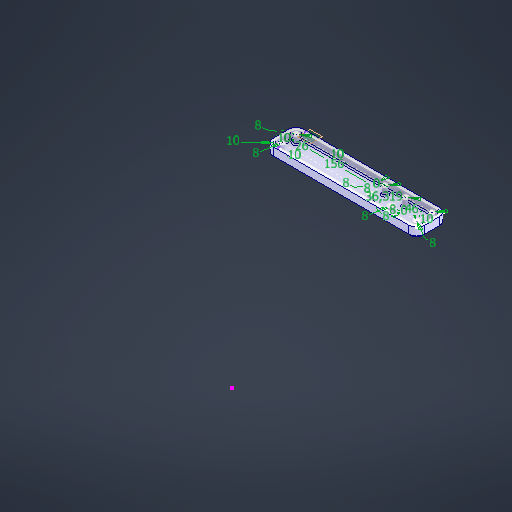
# Autodesk Inventor part: seitliche_Abdeckung_Kabel
Saved by Autodesk Inventor 2026.1 (Build 301233020, 233B)
## iProperties
Created: 2026-03-07
Part Number: seitliche_Abdeckung_Kabel
Material: Generisch
Document SubType Name: Modeling
Designer: neume
Density: 1 g/cm^3
Appearance: Vorgabe
Source: unknown
Author: neume
Autodesk Inventor part; units mm, degrees
ref_plane "YZ Plane" through (0, 0, 0) normal (1, 0, 0) x (0, 1, 0)
ref_plane "XZ Plane" through (0, 0, 0) normal (0, 1, 0) x (-1, 0, 0)
ref_plane "XY Plane" through (0, 0, 0) normal (0, 0, 1) x (1, 0, 0)
ref_plane "Arbeitsebene1" through (-314.8829, -4.3915, -452.3743) normal (0, -1, 0) x (1, 0, 0)
sketch "Skizze1" plane through (-314.8829, -4.3915, -452.3743) normal (0, -1, 0) x (1, 0, 0)
  line L0 (-16.319, 44) -> (222, 44)
  line L1 (232, 34) -> (232, 8)
  line L2 (222, -2) -> (-16.319, -2)
  line L3 (-16.319, 34) -> (139.681, 34) construction
  line L4 (139.681, 34) -> (139.681, 8) construction
  line L5 (139.681, 8) -> (-16.319, 8) construction
  line L6 (-16.319, 8) -> (-16.319, 34) construction
  circle A0 centre (-16.319, 34) radius 4
  circle A1 centre (-16.319, 8) radius 4
  circle A2 centre (139.681, 8) radius 4
  circle A3 centre (139.681, 34) radius 4
  line L7 (176, 34) -> (222, 34) construction
  line L8 (222, 34) -> (222, 8) construction
  line L9 (222, 8) -> (176, 8) construction
  line L10 (176, 8) -> (176, 34) construction
  circle A4 centre (176, 34) radius 4
  circle A5 centre (176, 8) radius 4
  circle A6 centre (222, 8) radius 4
  circle A7 centre (222, 34) radius 4
  arc A8 (-16.319, 44) -> (-26.319, 34) centre (-16.319, 34) ccw
  arc A9 (-26.319, 8) -> (-16.319, -2) centre (-16.319, 8) ccw
  arc A10 (222, -2) -> (232, 8) centre (222, 8) ccw
  arc A11 (232, 34) -> (222, 44) centre (222, 34) ccw
  line L11 (-26.319, 34) -> (-26.319, 8)
  point P0 (314.8829, 452.3743)
  point P1 (-10, 44)
  point P2 (232, -2)
  point P3 (232, 44)
  point P4 (-10, -2)
  dimension "d3" = 8
  dimension "d4" = 8
  dimension "d5" = 8
  dimension "d6" = 8
  dimension "d8" = 10
  dimension "d9" = 26
  dimension "d10" = 156
  dimension "d11" = 8
  dimension "d12" = 8
  dimension "d13" = 8
  dimension "d14" = 8
  dimension "d16" = 46
  dimension "d17" = 10
  dimension "d18" = 0
  dimension "d19" = 0
  dimension "d20" = 36.319
  dimension "d21" = 10
  dimension "d22" = 10
  dimension "d82" = 10
  constraints: 24 end point, 12 centre point, 8 coincident, 8 point on circle, 8 tangent, 6 point on line, 5 parallel, 4 horizontal, 3 equal radius, 3 perpendicular, 2 vertical
  measures "d3" diameter of A0
  measures "d4" diameter of A1
  measures "d5" diameter of A2
  measures "d6" diameter of A3
  measures "d8" distance between parallel lines of L0 L3
  measures "d9" distance between parallel lines of L3 L5
  measures "d10" distance between parallel lines of L4 L6
  measures "d11" diameter of A4
  measures "d12" diameter of A5
  measures "d13" diameter of A6
  measures "d14" diameter of A7
  measures "d16" distance between parallel lines of L8 L10
  measures "d17" distance between parallel lines of L1 L8
  measures "d18" distance between parallel lines of L3 L7
  measures "d19" distance between parallel lines of L9 L5
  measures "d20" distance between parallel lines of L4 L10
  measures "d21" distance between parallel lines of L2 L5
  measures "d22" radius of A8
  measures "d82" distance between parallel lines of L6 L11
extrude "Extrusion1" add sketch "Skizze1" along normal blind 14 contours L0 A11 L1 A10 L2 A9 L11 A8 | A0 | A1 | A2 | A3 | A4 | A5 | A6 | A7
chamfer "Fasen5" distance 2 angle 45 8 edges at (-85.8119, -18.3915, -451.4453) (-82.8829, -18.3915, -431.3743) (-85.8119, -18.3915, -411.3032) (-212.0424, -18.3915, -408.3743) (-338.273, -18.3915, -411.3032) (-341.2019, -18.3915, -431.3743) (-338.273, -18.3915, -451.4453) (-212.0424, -18.3915, -454.3743)
shell "Wandung8" thickness 4 outward yes removed faces 1 at (-251.7623, -4.3915, -439.0409)
extrude "Extrusion3" add sketch "Skizze1" along normal blind 14 contours A0 | A1 | A2 | A3 | A4 | A5 | A6 | A7
hole "Bohrung1" at (-92.8829, -4.3915, -418.3743) direction (0, -1, 0) diameter 3.2 end through all
hole "Bohrung2" at (-138.8829, -4.3915, -418.3743) at (-175.2019, -4.3915, -418.3743) at (-138.8829, -4.3915, -444.3743) at (-92.8829, -4.3915, -444.3743) at (-175.2019, -4.3915, -444.3743) at (-331.2019, -4.3915, -418.3743) at (-331.2019, -4.3915, -444.3743) direction (0, -1, 0) diameter 3.2 end through all
chamfer "Fasen6" distance 2 angle 45 8 edges at (-138.8829, -22.3915, -445.9743) (-92.8829, -22.3915, -445.9743) (-92.8829, -22.3915, -419.9743) (-138.8829, -22.3915, -419.9743) (-175.2019, -22.3915, -445.9743) (-175.2019, -22.3915, -419.9743) (-331.2019, -22.3915, -419.9743) (-331.2019, -22.3915, -445.9743)
chamfer "Fasen7" distance 2 angle 45 8 edges at (-96.8829, -18.3915, -418.3743) (-96.8829, -18.3915, -444.3743) (-142.8829, -18.3915, -444.3743) (-179.2019, -18.3915, -444.3743) (-142.8829, -18.3915, -418.3743) (-179.2019, -18.3915, -418.3743) (-335.2019, -18.3915, -418.3743) (-335.2019, -18.3915, -444.3743)
